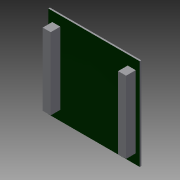
# Autodesk Inventor part: SFE-Host01
Saved by Autodesk Inventor 2013 (Build 170138000, 138)
## iProperties
Created: 2014-04-13
Part Number: SFE-Host01
Material: PCB(1)
Document SubType Name: Modeling
Designer: spichelh
Density: 1 g/cm^3
Author: spichelh
Autodesk Inventor part; units mm, degrees
ref_plane "YZ Plane" through (0, 0, 0) normal (1, 0, 0) x (0, 1, 0)
ref_plane "XZ Plane" through (0, 0, 0) normal (0, 1, 0) x (-1, 0, 0)
ref_plane "XY Plane" through (0, 0, 0) normal (0, 0, 1) x (1, 0, 0)
sketch "Sketch1" plane through (0, 0, 0) normal (0, 0, 1) x (1, 0, 0)
  line L0 (-28.575, -28.575) -> (28.575, -28.575)
  line L1 (28.575, -28.575) -> (28.575, 28.575)
  line L2 (28.575, 28.575) -> (-28.575, 28.575)
  line L3 (-28.575, 28.575) -> (-28.575, -28.575)
  line L4 (-28.575, -28.575) -> (28.575, 28.575) construction
  line L5 (28.575, -28.575) -> (-28.575, 28.575) construction
  line L6 (-28.575, 0) -> (28.575, 0) construction
  line L7 (0, 28.575) -> (0, -28.575) construction
  point P0 (0, 0)
  dimension "d2" = 57.15
  dimension "d4" = 57.15
  constraints: 16 end point, 6 midpoint, 2 parallel, 1 horizontal, 1 perpendicular
  measures "d2" distance of L1.end L2.end
  measures "d4" distance of L0.end L1.end
extrude "Extrusion1" add sketch "Sketch1" along normal blind 1
sketch "Sketch4" plane through (0, 0, 1) normal (0, 0, 1) x (1, 0, 0)
  line L0 (28.575, -28.575) -> (28.575, 28.575) projected
  line L1 (-28.575, 28.575) -> (-28.575, -28.575) projected
  line L2 (0, 0) -> (0, 45.0767)
  line L3 (21.035, 22.5) -> (26.035, 22.5)
  line L4 (26.035, 22.5) -> (26.035, -22.5)
  line L5 (26.035, -22.5) -> (21.035, -22.5)
  line L6 (21.035, -22.5) -> (21.035, 22.5)
  line L7 (-21.035, 22.5) -> (-26.035, 22.5)
  line L8 (-26.035, 22.5) -> (-26.035, -22.5)
  line L9 (-26.035, -22.5) -> (-21.035, -22.5)
  line L10 (-21.035, -22.5) -> (-21.035, 22.5)
  dimension "d21" = 2.54
  dimension "d22" = 45
  dimension "d23" = 5
  dimension "d24" = 22.5
  constraints: 18 end point, 4 symmetric about line, 3 parallel, 1 horizontal, 1 perpendicular
  measures "d21" distance between parallel lines of L4 L0
  measures "d22" distance between parallel lines of L5 L3
  measures "d23" distance between parallel lines of L4 L6
  measures "d24" distance from line of L2.start L3
extrude "Extrusion4" add sketch "Sketch4" along normal blind 6
body "Solid1"
